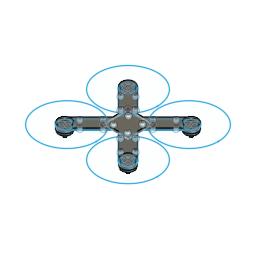
droneTest (Autodesk Fusion 360 design; units mm, degrees)
part number: 2026-03-09-17-57-18-484
Autodesk Fusion 360 part; units mm, degrees
sketch "Sketch1" plane through (0, 0, 0) normal (0, 0, 1) x (1, 0, 0)
  line L0 (5.1145, 0) -> (50, 0)
  line L1 (55, -5) -> (55, -50)
  line L2 (50, -55) -> (5, -55)
  line L3 (0, -50) -> (0, -5.1145)
  circle A0 centre (12, -11) radius 2
  circle A1 centre (43, -11) radius 2
  circle A2 centre (12, -44) radius 2
  circle A3 centre (43, -44) radius 2
  line L4 (0, -5.1145) -> (0, 0)
  line L5 (0, 0) -> (5.1145, 0)
  line L6 (50, 0) -> (55, 0)
  line L7 (55, 0) -> (55, -5)
  line L8 (50, -55) -> (55, -55)
  line L9 (55, -55) -> (55, -50)
  line L10 (0, -50) -> (0, -55)
  line L11 (0, -55) -> (5, -55)
  line L12 (0, -21.2132) -> (21.2132, 0)
  line L13 (21.2132, 0) -> (-31.8198, 53.033)
  line L14 (-31.8198, 53.033) -> (-53.033, 31.8198)
  line L15 (-53.033, 31.8198) -> (0, -21.2132)
  line L16 (21.2132, -55) -> (0, -33.7868)
  line L17 (0, -33.7868) -> (-53.033, -86.8198)
  line L18 (-53.033, -86.8198) -> (-31.8198, -108.033)
  line L19 (-31.8198, -108.033) -> (21.2132, -55)
  line L20 (33.7868, -55) -> (55, -33.7868)
  line L21 (55, -33.7868) -> (108.033, -86.8198)
  line L22 (108.033, -86.8198) -> (86.8198, -108.033)
  line L23 (86.8198, -108.033) -> (33.7868, -55)
  line L24 (33.7868, 0) -> (55, -21.2132)
  line L25 (55, -21.2132) -> (108.033, 31.8198)
  line L26 (108.033, 31.8198) -> (86.8198, 53.033)
  line L27 (86.8198, 53.033) -> (33.7868, 0)
  circle A4 centre (-40, -95) radius 64.77
  circle A5 centre (95, -95) radius 64.77
  circle A6 centre (-40, 40) radius 64.77
  circle A7 centre (95, 40) radius 64.77
  circle A8 centre (63.2024, -46.7976) radius 2
  circle A9 centre (46.7976, -63.2024) radius 2
  circle A10 centre (72.7831, -88.8345) radius 2
  circle A11 centre (88.8345, -72.7831) radius 2
  circle A12 centre (97.4264, -97.4264) radius 8
  circle A13 centre (97.4264, -89.4264) radius 2
  circle A14 centre (105.4264, -97.4264) radius 2
  circle A15 centre (97.4264, -105.4264) radius 2
  circle A16 centre (89.4264, -97.4264) radius 2
  circle A17 centre (97.4264, -97.4264) radius 13.75
  circle A18 centre (97.4264, -97.4264) radius 15
  circle A19 centre (-42.4264, -97.4264) radius 8
  circle A20 centre (-42.4264, -105.4264) radius 2
  circle A21 centre (-50.4264, -97.4264) radius 2
  circle A22 centre (-42.4264, -89.4264) radius 2
  circle A23 centre (-34.4264, -97.4264) radius 2
  circle A24 centre (-42.4264, -97.4264) radius 13.75
  circle A25 centre (-42.4264, -97.4264) radius 15
  circle A26 centre (-42.4264, 42.4264) radius 8
  circle A27 centre (-50.4264, 42.4264) radius 2
  circle A28 centre (-42.4264, 50.4264) radius 2
  circle A29 centre (-34.4264, 42.4264) radius 2
  circle A30 centre (-42.4264, 34.4264) radius 2
  circle A31 centre (-42.4264, 42.4264) radius 15
  circle A32 centre (-42.4264, 42.4264) radius 13.75
  circle A33 centre (97.4264, 42.4264) radius 15
  circle A34 centre (97.4264, 42.4264) radius 13.75
  circle A35 centre (97.4264, 42.4264) radius 8
  circle A36 centre (97.4264, 50.4264) radius 2
  circle A37 centre (105.4264, 42.4264) radius 2
  circle A38 centre (97.4264, 34.4264) radius 2
  circle A39 centre (89.4264, 42.4264) radius 2
  circle A40 centre (63.2024, -8.2024) radius 2
  circle A41 centre (46.7976, 8.2024) radius 2
  circle A42 centre (88.8345, 17.7831) radius 2
  circle A43 centre (72.7831, 33.8345) radius 2
  circle A44 centre (8.2024, 8.2024) radius 2
  circle A45 centre (-8.2024, -8.2024) radius 2
  circle A46 centre (-17.8538, 33.9052) radius 2
  circle A47 centre (-33.9052, 17.8538) radius 2
  circle A48 centre (-8.2024, -46.7976) radius 2
  circle A49 centre (8.2024, -63.2024) radius 2
  circle A50 centre (-33.8345, -72.7831) radius 2
  circle A51 centre (-17.7831, -88.8345) radius 2
  circle A52 centre (97.4264, -105.4264) radius 3
  circle A53 centre (89.4264, -97.4264) radius 3
  circle A54 centre (97.4264, -89.4264) radius 3
  circle A55 centre (105.4264, -97.4264) radius 3
  circle A56 centre (105.4264, 42.4264) radius 3
  circle A57 centre (97.4264, 50.4264) radius 3
  circle A58 centre (89.4264, 42.4264) radius 3
  circle A59 centre (97.4264, 34.4264) radius 3
  circle A60 centre (-34.4264, 42.4264) radius 3
  circle A61 centre (-42.4264, 50.4264) radius 3
  circle A62 centre (-50.4264, 42.4264) radius 3
  circle A63 centre (-42.4264, 34.4264) radius 3
  circle A64 centre (-42.4264, -89.4264) radius 3
  circle A65 centre (-50.4264, -97.4264) radius 3
  circle A66 centre (-34.4264, -97.4264) radius 3
  circle A67 centre (-42.4264, -105.4264) radius 3
  point P0 (55, 0)
  point P1 (0, -55)
  dimension "d1" = 55
  dimension "d2" = 55
  dimension "d7" = 4
  dimension "d8" = 12
  dimension "d9" = 11
  dimension "d11" = 4
  dimension "d12" = 12
  dimension "d13" = 11
  dimension "d14" = 4
  dimension "d15" = 11
  dimension "d16" = 12
  dimension "d17" = 4
  dimension "d18" = 12
  dimension "d19" = 11
  dimension "d22" = 75
  dimension "d23" = 30
  dimension "d24" = 75
  dimension "d25" = 30
  dimension "d26" = 75
  dimension "d27" = 30
  dimension "d28" = 75
  dimension "d29" = 30
  dimension "d31" = 129.54
  dimension "d32" = 129.54
  dimension "d33" = 129.54
  dimension "d34" = 129.54
  dimension "d35" = 4
  dimension "d36" = 3.4
  dimension "d37" = 15
  dimension "d39" = 4
  dimension "d40" = 3.4
  dimension "d41" = 15
  dimension "d42" = 4
  dimension "d43" = 36.5
  dimension "d44" = 3.65
  dimension "d45" = 4
  dimension "d46" = 3.65
  dimension "d49" = 16
  dimension "d52" = 4
  dimension "d53" = 4
  dimension "d54" = 4
  dimension "d55" = 4
  dimension "d56" = 27.5
  dimension "d57" = 16
  dimension "d58" = 4
  dimension "d59" = 4
  dimension "d60" = 4
  dimension "d61" = 4
  dimension "d62" = 27.5
  dimension "d63" = 30
  dimension "d64" = 16
  dimension "d65" = 4
  dimension "d66" = 4
  dimension "d67" = 4
  dimension "d68" = 4
  dimension "d69" = 30
  dimension "d70" = 27.5
  dimension "d71" = 30
  dimension "d72" = 27.5
  dimension "d73" = 16
  dimension "d74" = 4
  dimension "d75" = 4
  dimension "d76" = 4
  dimension "d77" = 4
  dimension "d78" = 36.5
  dimension "d79" = 4
  dimension "d80" = 3.4
  dimension "d81" = 15
  dimension "d82" = 4
  dimension "d83" = 3.4
  dimension "d84" = 15
  dimension "d85" = 4
  dimension "d86" = 3.65
  dimension "d87" = 36.5
  dimension "d88" = 4
  dimension "d89" = 3.65
  dimension "d90" = 36.5
  dimension "d91" = 4
  dimension "d92" = 4
  dimension "d93" = 4
  dimension "d94" = 4
  dimension "d95" = 15
  dimension "d96" = 15
  dimension "d101" = 36.6
  dimension "d102" = 36.6
  dimension "d103" = 4
  dimension "d104" = 4
  dimension "d105" = 4
  dimension "d106" = 4
  dimension "d107" = 3.4
  dimension "d108" = 15
  dimension "d109" = 15
  dimension "d110" = 3.4
  dimension "d111" = 3.65
  dimension "d112" = 3.65
  dimension "d113" = 36.5
  dimension "d114" = 36.5
  dimension "d115" = 23.2
  dimension "d116" = 3.4
  dimension "d117" = 3.4
  dimension "d118" = 22.7
  dimension "d119" = 3.65
  dimension "d120" = 3.65
  dimension "d169" = 6
  dimension "d170" = 6
  dimension "d171" = 6
  dimension "d172" = 6
  dimension "d191" = 6
  dimension "d192" = 6
  dimension "d193" = 6
  dimension "d194" = 6
  dimension "d195" = 6
  dimension "d196" = 6
  dimension "d197" = 6
  dimension "d198" = 6
  dimension "d199" = 6
  dimension "d200" = 6
  dimension "d201" = 6
  dimension "d202" = 6
  constraint horizontal L0
  constraint vertical L1
  constraint horizontal L2
  constraint vertical L3
  constraint coincident L4.end L5.start
  constraint coincident L4.end L0
  constraint coincident L4.end L3
  constraint coincident P0 L1
  constraint coincident P0 L0
  constraint coincident P1 L2
  constraint coincident P1 L3
  constraint coincident P0 L6.end
  constraint parallel L2 L8
  constraint coincident P1 L10.end
  constraint perpendicular L12 L13
  constraint parallel L12 L14
  constraint parallel L13 L15
  constraint coincident L0 L12.end
  constraint coincident L3 L12.start
  constraint perpendicular L16 L17
  constraint parallel L16 L18
  constraint parallel L17 L19
  constraint coincident L3 L16.end
  constraint coincident L2 L16.start
  constraint perpendicular L20 L21
  constraint parallel L20 L22
  constraint parallel L21 L23
  constraint coincident L1 L20.end
  constraint coincident L2 L20.start
  constraint perpendicular L24 L25
  constraint parallel L24 L26
  constraint parallel L25 L27
  constraint coincident L1 L24.end
  constraint coincident L0 L24.start
  constraint midpoint L22 A12.centre
  constraint coincident A12 A13.centre
  constraint coincident A12 A14.centre
  constraint coincident A12 A15.centre
  constraint coincident A12 A16.centre
  constraint concentric A12 A17
  constraint concentric A12 A18
  constraint coincident L22.end A18
  constraint midpoint L18 A19.centre
  constraint coincident A19 A20.centre
  constraint coincident A19 A21.centre
  constraint coincident A19 A22.centre
  constraint coincident A19 A23.centre
  constraint concentric A19 A24
  constraint concentric A24 A25
  constraint midpoint L14 A26.centre
  constraint coincident A26 A27.centre
  constraint coincident A26 A28.centre
  constraint coincident A26 A29.centre
  constraint coincident A26 A30.centre
  constraint concentric A26 A31
  constraint concentric A31 A32
  constraint midpoint L26 A33.centre
  constraint concentric A33 A34
  constraint concentric A34 A35
  constraint coincident A35 A36.centre
  constraint coincident A35 A37.centre
  constraint coincident A35 A38.centre
  constraint coincident A35 A39.centre
  constraint concentric A15 A52
  constraint concentric A16 A53
  constraint concentric A13 A54
  constraint concentric A14 A55
  constraint concentric A37 A56
  constraint concentric A36 A57
  constraint concentric A39 A58
  constraint concentric A38 A59
  constraint concentric A29 A60
  constraint concentric A28 A61
  constraint concentric A27 A62
  constraint concentric A30 A63
  constraint concentric A22 A64
  constraint concentric A21 A65
  constraint concentric A23 A66
  constraint concentric A20 A67
  measures "d1" distance of L4.end P0
  measures "d2" distance of L4.end L10.end
  measures "d7" diameter of A0
  measures "d8" distance of L3 A0.centre
  measures "d9" distance of L0 A0.centre
  measures "d11" diameter of A1
  measures "d12" distance of L1 A1.centre
  measures "d13" distance of L0 A1.centre
  measures "d14" diameter of A2
  measures "d15" distance of L2 A2.centre
  measures "d16" distance of L3 A2.centre
  measures "d17" diameter of A3
  measures "d18" distance of L1 A3.centre
  measures "d19" distance of L2 A3.centre
  measures "d22" distance of L12.start L14.end
  measures "d23" distance of L13 L15
  measures "d24" distance of L16.start L18.end
  measures "d25" distance of L17 L19
  measures "d26" distance of L20.start L22.end
  measures "d27" distance of L21 L23
  measures "d28" distance of L24.start L26.end
  measures "d29" distance of L25 L27
  measures "d31" diameter of A4
  measures "d32" diameter of A5
  measures "d33" diameter of A6
  measures "d34" diameter of A7
  measures "d35" diameter of A8
  measures "d36" distance of L21 A8.centre
  measures "d37" distance of L20 A8.centre
  measures "d39" diameter of A9
  measures "d40" distance of L23 A9.centre
  measures "d41" distance of L20 A9.centre
  measures "d42" diameter of A10
  measures "d43" distance of A9.centre A10.centre
  measures "d44" distance of L23 A10.centre
  measures "d45" diameter of A11
  measures "d46" distance of L21 A11.centre
  measures "d49" diameter of A12
  measures "d52" diameter of A13
  measures "d53" diameter of A14
  measures "d54" diameter of A15
  measures "d55" diameter of A16
  measures "d56" diameter of A17
  measures "d57" diameter of A19
  measures "d58" diameter of A20
  measures "d59" diameter of A21
  measures "d60" diameter of A22
  measures "d61" diameter of A23
  measures "d62" diameter of A24
  measures "d63" diameter of A25
  measures "d64" diameter of A26
  measures "d65" diameter of A27
  measures "d66" diameter of A28
  measures "d67" diameter of A29
  measures "d68" diameter of A30
  measures "d69" diameter of A31
  measures "d70" diameter of A32
  measures "d71" diameter of A33
  measures "d72" diameter of A34
  measures "d73" diameter of A35
  measures "d74" diameter of A36
  measures "d75" diameter of A37
  measures "d76" diameter of A38
  measures "d77" diameter of A39
  measures "d78" distance of A8.centre A11.centre
  measures "d79" diameter of A40
  measures "d80" distance of L25 A40.centre
  measures "d81" distance of L24 A40.centre
  measures "d82" diameter of A41
  measures "d83" distance of L27 A41.centre
  measures "d84" distance of L24 A41.centre
  measures "d85" diameter of A42
  measures "d86" distance of L25 A42.centre
  measures "d87" distance of A40.centre A42.centre
  measures "d88" diameter of A43
  measures "d89" distance of L27 A43.centre
  measures "d90" distance of A41.centre A43.centre
  measures "d91" diameter of A44
  measures "d92" diameter of A45
  measures "d93" diameter of A46
  measures "d94" diameter of A47
  measures "d95" distance of L12 A44.centre
  measures "d96" distance of L12 A45.centre
  measures "d101" distance of A45.centre A47.centre
  measures "d102" distance of A44.centre A46.centre
  measures "d103" diameter of A48
  measures "d104" diameter of A49
  measures "d105" diameter of A50
  measures "d106" diameter of A51
  measures "d107" distance of L17 A48.centre
  measures "d108" distance of L16 A48.centre
  measures "d109" distance of L16 A49.centre
  measures "d110" distance of L19 A49.centre
  measures "d111" distance of L19 A51.centre
  measures "d112" distance of L17 A50.centre
  measures "d113" distance of A48.centre A50.centre
  measures "d114" distance of A49.centre A51.centre
  measures "d115" distance of A44.centre A45.centre
  measures "d116" distance of L15 A45.centre
  measures "d117" distance of L13 A44.centre
  measures "d118" distance of A46.centre A47.centre
  measures "d119" distance of L15 A47.centre
  measures "d120" distance of L13 A46.centre
  measures "d169" diameter of A52
  measures "d170" diameter of A53
  measures "d171" diameter of A54
  measures "d172" diameter of A55
  measures "d191" diameter of A56
  measures "d192" diameter of A57
  measures "d193" diameter of A58
  measures "d194" diameter of A59
  measures "d195" diameter of A60
  measures "d196" diameter of A61
  measures "d197" diameter of A62
  measures "d198" diameter of A63
  measures "d199" diameter of A64
  measures "d200" diameter of A65
  measures "d201" diameter of A66
  measures "d202" diameter of A67
extrude "Extrude1" add sketch "Sketch1" along normal blind 3 contours L0 L3 A0 L12 A6 | L0 L1 L2 L3 A0 A1 A2 A3 L12 L16 L20 L24 | L0 L13 A6 | L0 L27 A7 | L0 L1 A1 L24 A7 | L0 L3 L4 L5 A6 | L0 L3 L4 L5 L13 L15 A6 A31 | L0 L1 L6 L7 L25 L27 A7 A33 | L0 L1 L6 L7 A7 | L3 L15 A6 | L14 A31 A32 | L14 A31 A32 | L1 L25 A7 | L26 A33 A34 | L26 A33 A34 | L14 A26 A32 A60 A63 | L14 A26 A32 A61 A62 | L26 A34 A35 A56 A57 | L26 A34 A35 A58 A59 | L2 L3 A2 L16 A4 | L3 L17 A4 | L14 A26 A60 A63 | L14 A26 A61 A62 | L1 L21 A5 | L1 L2 A3 L20 A5 | L26 A35 A56 A57 | L26 A35 A58 A59 | L2 L3 L10 L11 A4 | L2 L3 L10 L11 L17 L19 A4 A25 | A26 A29 A60 | A26 A29 A60 | A26 A28 A61 | A26 A28 A61 | L1 L2 L8 L9 L21 L23 A5 A18 | L1 L2 L8 L9 A5 | A35 A36 A57 | A35 A36 A57 | A35 A39 A58 | A35 A39 A58 | L2 L19 A4 | L18 A24 A25 | L18 A24 A25 | A26 A27 A62 | A26 A27 A62 | A26 A30 A63 | A26 A30 A63 | L2 L23 A5 | L22 A17 A18 | L22 A17 A18 | A35 A38 A59 | A35 A38 A59 | A35 A37 A56 | A35 A37 A56 | L18 A19 A24 A64 A66 | L18 A19 A24 A65 A67 | L22 A12 A17 A52 A55 | L22 A12 A17 A53 A54 | L18 A19 A64 A66 | L18 A19 A65 A67 | L22 A12 A52 A55 | L22 A12 A53 A54 | A19 A22 A64 | A19 A22 A64 | A19 A21 A65 | A19 A21 A65 | A12 A14 A55 | A12 A14 A55 | A12 A13 A54 | A12 A13 A54 | A19 A20 A67 | A19 A20 A67 | A19 A23 A66 | A19 A23 A66 | A12 A16 A53 | A12 A16 A53 | A12 A15 A52 | A12 A15 A52 makes body 1
extrude "Extrude2" add 1 faces at (22.9395, -22.5239, 3) along direction (0, 0, 1) blind 1 on bodies 1 bodies 1
extrude "Extrude3" cut sketch "Sketch1" along normal blind 10 contours L14 A26 A32 A60 A63 | L14 A26 A32 A61 A62 | L14 A26 A60 A63 | L14 A26 A61 A62 | A26 A29 A60 | A26 A29 A60 | A26 A28 A61 | A26 A28 A61 | A26 A27 A62 | A26 A27 A62 | A26 A30 A63 | A26 A30 A63 bodies 1
extrude "Extrude4" add sketch "Sketch1" along normal blind 10 contours L14 A26 A32 A60 A63 | L14 A26 A32 A61 A62 | L14 A26 A60 A63 | L14 A26 A61 A62 | A26 A29 A60 | A26 A29 A60 | A26 A28 A61 | A26 A28 A61 | A26 A27 A62 | A26 A27 A62 | A26 A30 A63 | A26 A30 A63 bodies 1
extrude "Extrude5" cut sketch "Sketch1" along normal blind 10 contours L26 A34 A35 A56 A57 | L26 A34 A35 A58 A59 | L26 A35 A56 A57 | L26 A35 A58 A59 | A35 A36 A57 | A35 A36 A57 | A35 A39 A58 | A35 A39 A58 | A35 A38 A59 | A35 A38 A59 | A35 A37 A56 | A35 A37 A56 | L18 A19 A24 A64 A66 | L18 A19 A24 A65 A67 | L22 A12 A17 A52 A55 | L22 A12 A17 A53 A54 | L18 A19 A64 A66 | L18 A19 A65 A67 | L22 A12 A52 A55 | L22 A12 A53 A54 | A19 A22 A64 | A19 A22 A64 | A19 A21 A65 | A19 A21 A65 | A12 A14 A55 | A12 A14 A55 | A12 A13 A54 | A12 A13 A54 | A19 A20 A67 | A19 A20 A67 | A19 A23 A66 | A19 A23 A66 | A12 A16 A53 | A12 A16 A53 | A12 A15 A52 | A12 A15 A52 bodies 1
extrude "Extrude6" add sketch "Sketch1" along normal blind 10 contours L26 A34 A35 A56 A57 | L26 A34 A35 A58 A59 | L26 A35 A56 A57 | L26 A35 A58 A59 | A35 A36 A57 | A35 A36 A57 | A35 A39 A58 | A35 A39 A58 | A35 A38 A59 | A35 A38 A59 | A35 A37 A56 | A35 A37 A56 | L18 A19 A24 A64 A66 | L18 A19 A24 A65 A67 | L22 A12 A17 A52 A55 | L22 A12 A17 A53 A54 | L18 A19 A64 A66 | L18 A19 A65 A67 | L22 A12 A52 A55 | L22 A12 A53 A54 | A19 A22 A64 | A19 A22 A64 | A19 A21 A65 | A19 A21 A65 | A12 A14 A55 | A12 A14 A55 | A12 A13 A54 | A12 A13 A54 | A19 A20 A67 | A19 A20 A67 | A19 A23 A66 | A19 A23 A66 | A12 A16 A53 | A12 A16 A53 | A12 A15 A52 | A12 A15 A52 bodies 1
extrude "Extrude7" cut 4 faces at (97.346, 40.4215, 10) (-42.5068, 44.4313, 10) (-42.346, -95.4215, 10) (97.346, -99.4313, 10) along direction (0, 0, -1) blind 5 on bodies 1 bodies 1
extrude "Extrude8" add 1 faces at (97.346, -99.4313, 5) along direction (0, 0, -1) blind 6 on bodies 1 bodies 1
extrude "Extrude9" add 1 faces at (97.346, -99.4313, -1) along direction (0, 0, 1) blind 2 on bodies 1 bodies 1
extrude "Extrude10" add 1 faces at (97.346, -99.4313, -1) along direction (0, 0, -1) blind 2 on bodies 1 bodies 1
extrude "Extrude11" add sketch "Sketch1" against normal blind 7 contours L22 A12 A52 A55 | L22 A12 A53 A54 | A12 A14 A55 | A12 A13 A54 | A12 A16 A53 | A12 A15 A52 | A12 A14 | A12 A13 | A12 A16 | A12 A15 picked at (104.6818, -99.8582) picked at (99.8582, -90.171) picked at (90.1642, -99.8605) picked at (99.8582, -104.6818) picked at (104.7781, -97.839) picked at (96.813, -90.0523) picked at (90.0523, -96.813) picked at (96.813, -104.8005) bodies 1
extrude "Extrude12" add sketch "Sketch1" against normal blind 5 contours A12 A14 | A12 A13 | A12 A16 | A12 A15 picked at (106.0247, -97.9232) picked at (98.0975, -88.8726) picked at (88.8675, -96.764) picked at (98.0975, -105.9803) bodies 1
extrude "Extrude13" add sketch "Sketch1" against normal blind 3 contours L26 A34 A35 A56 A57 | L26 A34 A35 A58 A59 | A35 A36 A57 | A35 A39 A58 | A35 A38 A59 | A35 A37 A56 picked at (94.9952, 50.4291) picked at (89.4207, 44.8573) picked at (94.9952, 34.4237) picked at (105.428, 39.9955) bodies 1
extrude "Extrude14" add sketch "Sketch1" against normal blind 6 contours A35 A36 | A35 A39 | A35 A38 | A35 A37 picked at (98.0975, 50.9803) picked at (88.8675, 41.764) picked at (98.0975, 33.8726) picked at (106.0247, 41.9296) bodies 1
extrude "Extrude15" add sketch "Sketch1" against normal blind 7 contours L26 A35 A56 A57 | L26 A35 A58 A59 | A35 A36 A57 | A35 A39 A58 | A35 A38 A59 | A35 A37 A56 | A35 A36 | A35 A39 | A35 A38 | A35 A37 picked at (94.9947, 49.6818) picked at (90.1642, 39.9923) picked at (94.9947, 35.171) picked at (104.6818, 44.8582) picked at (98.0399, 49.8005) picked at (90.0523, 41.813) picked at (96.813, 35.0523) picked at (104.7781, 42.0138) bodies 1
extrude "Extrude16" add sketch "Sketch1" against normal blind 3 contours L14 A26 A32 A60 A63 | L14 A26 A32 A61 A62 | A26 A29 A60 | A26 A28 A61 | A26 A27 A62 | A26 A30 A63 picked at (-34.4248, 39.9955) picked at (-44.8576, 50.4291) picked at (-50.4321, 44.8573) picked at (-44.8576, 34.4237) bodies 1
extrude "Extrude17" add sketch "Sketch1" against normal blind 6 contours A26 A29 | A26 A28 | A26 A27 | A26 A30 picked at (-33.8281, 41.9296) picked at (-41.7553, 50.9803) picked at (-50.9853, 43.0888) picked at (-41.7553, 33.8726) bodies 1
extrude "Extrude18" add sketch "Sketch1" against normal blind 7 contours L14 A26 A60 A63 | L14 A26 A61 A62 | A26 A29 A60 | A26 A28 A61 | A26 A27 A62 | A26 A30 A63 | A26 A29 | A26 A28 | A26 A27 | A26 A30 picked at (-35.171, 39.9947) picked at (-44.8582, 49.6818) picked at (-49.6886, 44.8605) picked at (-44.8582, 35.171) picked at (-35.0747, 42.0138) picked at (-43.0399, 49.8005) picked at (-49.8005, 41.813) picked at (-43.0399, 35.0523) bodies 1
extrude "Extrude19" add sketch "Sketch1" against normal blind 3 contours L18 A19 A24 A64 A66 | L18 A19 A24 A65 A67 | A19 A22 A64 | A19 A21 A65 | A19 A20 A67 | A19 A23 A66 picked at (-44.8576, -89.4237) picked at (-50.4321, -94.9956) picked at (-44.8576, -105.4291) picked at (-34.4248, -99.8573) bodies 1
extrude "Extrude20" add sketch "Sketch1" against normal blind 6 contours A19 A22 | A19 A21 | A19 A20 | A19 A23 picked at (-41.7553, -88.8726) picked at (-50.9853, -96.764) picked at (-41.7553, -105.9803) picked at (-33.8281, -96.9296) bodies 1
extrude "Extrude21" add sketch "Sketch1" against normal blind 7 contours L18 A19 A64 A66 | L18 A19 A65 A67 | A19 A22 A64 | A19 A21 A65 | A19 A20 A67 | A19 A23 A66 | A19 A22 | A19 A21 | A19 A20 | A19 A23 picked at (-39.9947, -90.171) picked at (-49.6886, -99.8605) picked at (-44.8582, -104.6818) picked at (-35.171, -94.9947) picked at (-43.0399, -90.0523) picked at (-49.8005, -96.813) picked at (-43.0399, -104.8005) picked at (-35.0747, -97.839) bodies 1
extrude "Extrude22" add sketch "Sketch1" against normal blind 12 contours L22 A12 A17 A52 A55 | L22 A12 A17 A53 A54 | A12 A14 A55 | A12 A13 A54 | A12 A16 A53 | A12 A15 A52 picked at (105.428, -99.8573) picked at (94.9952, -89.4237) picked at (89.4207, -94.9956) picked at (94.9952, -105.4291) bodies 1
extrude "Extrude23" add sketch "Sketch1" against normal blind 7 contours L22 A17 A18 | L22 A17 A18 bodies 1
extrude "Extrude24" add sketch "Sketch1" against normal blind 7 contours L22 A17 A18 | L22 A17 A18 bodies 1
extrude "Extrude25" cut sketch "Sketch1" along normal blind -30 and the other way blind -6 contours A12 A14 A55 | A12 A14 A55 | A12 A14 | A12 A14 bodies 1
extrude "Extrude26" add sketch "Sketch1" along normal blind 5 contours A12 A14 A55 | A12 A14 A55 bodies 1
extrude "Extrude27" add 1 faces at (94.1257, -99.2826, -7) along direction (0, 0, -1) blind 11 on bodies 1 bodies 1
extrude "Extrude28" cut sketch "Sketch1" along normal mid plane 60 contours A12 A13 A54 | A12 A13 A54 | A12 A16 A53 | A12 A16 A53 | A12 A15 A52 | A12 A15 A52 | A12 A13 | A12 A13 | A12 A16 | A12 A16 | A12 A15 | A12 A15 bodies 1
extrude "Extrude29" add sketch "Sketch1" along normal blind 5 contours A12 A13 A54 | A12 A13 A54 | A12 A16 A53 | A12 A16 A53 | A12 A15 A52 | A12 A15 A52 bodies 1
extrude "Extrude30" add sketch "Sketch1" against normal blind 7 contours L26 A33 A34 | L26 A33 A34 bodies 1
extrude "Extrude31" add sketch "Sketch1" against normal blind 12 separate body contours L26 A34 A35 A56 A57 | L26 A34 A35 A58 A59 | A35 A36 A57 | A35 A39 A58 | A35 A38 A59 | A35 A37 A56 picked at (94.9952, 50.4291) picked at (89.4207, 44.8573) picked at (94.9952, 34.4237) picked at (105.428, 39.9955) makes body 2
extrude "Extrude32" add sketch "Sketch1" against normal blind 19 separate body contours L26 A35 A56 A57 | L26 A35 A58 A59 | A35 A36 A57 | A35 A39 A58 | A35 A38 A59 | A35 A37 A56 picked at (94.9947, 49.6818) picked at (90.1642, 39.9923) picked at (94.9947, 35.171) picked at (104.6818, 44.8582) makes body 3
extrude "Extrude33" cut sketch "Sketch1" along normal mid plane 40 contours A35 A36 A57 | A35 A36 A57 | A35 A39 A58 | A35 A39 A58 | A35 A38 A59 | A35 A38 A59 | A35 A37 A56 | A35 A37 A56 | A35 A36 | A35 A36 | A35 A39 | A35 A39 | A35 A38 | A35 A38 | A35 A37 | A35 A37 bodies 1 2 3
extrude "Extrude34" add sketch "Sketch1" along normal blind 5 contours A35 A36 A57 | A35 A36 A57 | A35 A39 A58 | A35 A39 A58 | A35 A38 A59 | A35 A38 A59 | A35 A37 A56 | A35 A37 A56 bodies 1 2 3
extrude "Extrude35" add sketch "Sketch1" against normal blind 19 separate body contours L14 A26 A60 A63 | L14 A26 A61 A62 makes body 4
extrude "Extrude36" add sketch "Sketch1" against normal blind 19 separate body contours L14 A26 A32 A60 A63 | L14 A26 A32 A61 A62 makes body 5
extrude "Extrude37" cut 1 faces at (-47.5438, 51.3129, -19) along direction (0, 0, 1) blind 7 on bodies 5 bodies 5
extrude "Extrude38" add sketch "Sketch1" against normal blind 7 contours L14 A31 A32 | L14 A31 A32 bodies 1 5
extrude "Extrude39" cut sketch "Sketch1" along normal mid plane 40 contours A26 A29 A60 | A26 A29 A60 | A26 A28 A61 | A26 A28 A61 | A26 A27 A62 | A26 A27 A62 | A26 A30 A63 | A26 A30 A63 | A26 A29 | A26 A29 | A26 A28 | A26 A28 | A26 A27 | A26 A27 | A26 A30 | A26 A30 bodies 1
extrude "Extrude40" add sketch "Sketch1" along normal blind 5 contours A26 A29 A60 | A26 A29 A60 | A26 A28 A61 | A26 A28 A61 | A26 A27 A62 | A26 A27 A62 | A26 A30 A63 | A26 A30 A63 bodies 1 4
extrude "Extrude41" add 1 faces at (-32.1932, -103.3174, -3) along direction (0, 0, -1) blind 9 on bodies 1 bodies 1
extrude "Extrude42" add sketch "Sketch1" against normal blind 7 contours L18 A24 A25 | L18 A24 A25 bodies 1
extrude "Extrude43" add 1 faces at (-41.6768, -95.0423, -7) along direction (0, 0, -1) blind 12 on bodies 1 bodies 1
extrude "Extrude44" cut sketch "Sketch1" along normal mid plane 40 contours A19 A22 A64 | A19 A22 A64 | A19 A21 A65 | A19 A21 A65 | A19 A20 A67 | A19 A20 A67 | A19 A23 A66 | A19 A23 A66 | A19 A22 | A19 A22 | A19 A21 | A19 A21 | A19 A20 | A19 A20 | A19 A23 | A19 A23 bodies 1
extrude "Extrude45" add sketch "Sketch1" along normal blind 5 contours A19 A22 A64 | A19 A22 A64 | A19 A21 A65 | A19 A21 A65 | A19 A20 A67 | A19 A20 A67 | A19 A23 A66 | A19 A23 A66 bodies 1
extrude "Extrude46" add 1 faces at (97.3766, -99.4283, 5) along direction (0, 0, 1) blind 1 on bodies 1 bodies 1
extrude "Extrude47" add 1 faces at (-42.346, -95.4215, 5) along direction (0, 0, 1) blind 1 on bodies 1 bodies 1
extrude "Extrude48" add 1 faces at (-42.3766, 44.4283, 5) along direction (0, 0, 1) blind 1 on bodies 1 bodies 1
extrude "Extrude49" add 1 faces at (97.4762, 40.4245, 5) along direction (0, 0, 1) blind 1 on bodies 1 bodies 1
